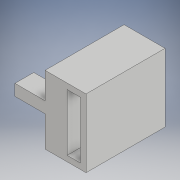
# Autodesk Inventor part: ShooterProto
Saved by Autodesk Inventor 2017 (Build 210142000, 142)
## iProperties
Created: 2017-05-20
Part Number: ShooterProto
Material: Generic
Document SubType Name: Modeling
Designer: User
Density: 1 g/cm^3
Appearance: Default
Author: User
Autodesk Inventor part; units mm, degrees
ref_plane "YZ Plane" through (0, 0, 0) normal (1, 0, 0) x (0, 1, 0)
ref_plane "XZ Plane" through (0, 0, 0) normal (0, 1, 0) x (-1, 0, 0)
ref_plane "XY Plane" through (0, 0, 0) normal (0, 0, 1) x (1, 0, 0)
sketch "Sketch1" plane through (0, 0, 0) normal (1, 0, 0) x (0, 1, 0)
  line L0 (0, 0) -> (230.2002, 0)
  line L1 (230.2002, 0) -> (230.2002, -138.176)
  line L2 (230.2002, -138.176) -> (0, -138.176)
  line L3 (0, -138.176) -> (0, 0)
  dimension "d0" = 230.2002
  dimension "d1" = 138.176
  constraints: 8 end point, 2 parallel, 1 horizontal, 1 perpendicular
  measures "d0" distance of L1.end L2.end
  measures "d1" distance of L0.end L1.end
extrude "Extrusion1" add sketch "Sketch1" along normal blind 266.7
sketch "Sketch2" plane through (266.7, 0, 0) normal (1, 0, 0) x (0, 0, -1)
  line L0 (0, 230.2002) -> (0, 0) projected
  line L1 (0, 0) -> (138.176, 0) projected
  line L2 (138.176, 0) -> (138.176, 230.2002) projected
  line L3 (138.176, 230.2002) -> (0, 230.2002) projected
  line L4 (19.05, 211.1502) -> (63.5, 211.1502)
  line L5 (63.5, 211.1502) -> (63.5, 19.05)
  line L6 (63.5, 19.05) -> (19.05, 19.05)
  line L7 (19.05, 19.05) -> (19.05, 211.1502)
  dimension "d4" = 19.05
  dimension "d5" = 63.5
  dimension "d7" = 19.05
  dimension "d17" = 19.05
  constraints: 8 end point, 2 parallel, 1 horizontal, 1 perpendicular
  measures "d4" distance between parallel lines of L0 L7
  measures "d5" distance between parallel lines of L5 L0
  measures "d7" distance between parallel lines of L1 L6
  measures "d17" distance between parallel lines of L3 L4
extrude "Extrusion2" cut sketch "Sketch2" against normal blind 266.7 contours L4 L5 L6 L7
sketch "Sketch3" plane through (0, 0, 0) normal (-1, 0, 0) x (0, 0, 1)
  line L0 (-19.05, 211.1502) -> (-19.05, 19.05) projected
  line L1 (-19.05, 19.05) -> (-63.5, 19.05) projected
  line L2 (-63.5, 19.05) -> (-63.5, 211.1502) projected
  line L3 (-63.5, 211.1502) -> (-19.05, 211.1502) projected
  line L4 (0, 0) -> (0, 230.2002) projected
  line L5 (0, 230.2002) -> (-138.176, 230.2002) projected
  line L6 (-138.176, 230.2002) -> (-138.176, 0) projected
  line L7 (-138.176, 0) -> (0, 0) projected
  line L8 (-138.176, 103.2002) -> (-239.776, 103.2002)
  line L9 (-239.776, 103.2002) -> (-239.776, 141.3002)
  line L10 (-239.776, 141.3002) -> (-138.176, 141.3002)
  line L11 (-138.176, 141.3002) -> (-138.176, 103.2002)
  dimension "d11" = 101.6
  dimension "d12" = 38.1
  dimension "d14" = 127
  constraints: 8 end point, 2 parallel, 1 horizontal, 1 perpendicular, 1 point on line
  measures "d11" distance of L9.end L10.end
  measures "d12" distance of L8.end L9.end
  measures "d14" distance between parallel lines of L5 L8
extrude "Extrusion3" add sketch "Sketch3" against normal blind 63.5 contours L8 L9 L10 L6
body "Solid1"
